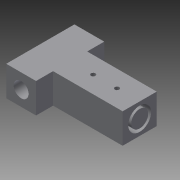
# Autodesk Inventor part: WagonHandleV01
Saved by Autodesk Inventor 2014 (Build 180170000, 170)
## iProperties
Created: 2013-11-15
Part Number: WagonHandleV01
Material: Generic
Document SubType Name: Modeling
Designer: steele
Density: 1 g/cm^3
Appearance: Default
Author: steele
Autodesk Inventor part; units mm, degrees
ref_plane "YZ Plane" through (0, 0, 0) normal (1, 0, 0) x (0, 1, 0)
ref_plane "XZ Plane" through (0, 0, 0) normal (0, 1, 0) x (-1, 0, 0)
sketch "Base for Part" plane through (0, 0, 0) normal (0, 0, 1) x (1, 0, 0)
  line L0 (0, 0) -> (148, 0) construction
  line L1 (0, 0) -> (0, 50.8)
  line L2 (0, 50.8) -> (44.45, 50.8)
  line L3 (148, -29.2) -> (148, 0)
  line L4 (44.45, 50.8) -> (44.45, 25.4)
  line L5 (44.45, 25.4) -> (148, 25.4)
  line L6 (148, 25.4) -> (148, 0)
  line L7 (0, 0) -> (0, -50.8)
  line L8 (0, -50.8) -> (44.45, -50.8)
  line L9 (44.45, -50.8) -> (44.45, -25.4)
  line L10 (44.45, -25.4) -> (148, -25.4)
  line L11 (148, -25.4) -> (148, 0)
  dimension "d0" = 148
  dimension "d1" = 50.8
  dimension "d2" = 44.45
  dimension "d3" = 25.4
  constraints: 24 end point, 4 perpendicular, 4 symmetric about line, 2 parallel
  measures "d0" distance of L0.start L0.end
  measures "d1" distance of L0.start L1.end
  measures "d2" distance of L1.end L2.end
  measures "d3" distance of L2.end L4.end
extrude "Extrusion of Base" add sketch "Base for Part" along normal blind 44.45
sketch "Sketch for 1 inch PVC" plane through (148, -25.4, 0) normal (1, 0, 0) x (0, 0, -1)
  line L0 (0, 50.8) -> (-44.45, 50.8) projected
  line L1 (-44.45, 0) -> (-44.45, 50.8) projected
  line L2 (0, 0) -> (-44.45, 0) projected
  line L3 (-44.45, 25.4) -> (0, 25.4) construction
  line L4 (-22.225, 50.8) -> (-22.225, 0) construction
  circle A0 centre (-22.225, 25.4) radius 12.6619
  circle A1 centre (-22.225, 25.4) radius 17.0434
  dimension "d6" = 34.0868
  dimension "d7" = 25.3238
  constraints: 4 end point, 4 midpoint, 2 centre point, 1 coincident, 1 parallel
  measures "d6" diameter of A1
  measures "d7" diameter of A0
extrude "Extrusion for 1 inch PVC" cut sketch "Sketch for 1 inch PVC" against normal blind 114.55
sketch "Sketch of Base Hole" plane through (0, -50.8, 0) normal (0, -1, 0) x (1, 0, 0)
  line L0 (44.45, 0) -> (0, 0) projected
  line L1 (44.45, 0) -> (44.45, 44.45) projected
  line L2 (0, 44.45) -> (44.45, 44.45) projected
  line L3 (0, 0) -> (0, 44.45) projected
  line L4 (0, 22.225) -> (44.45, 22.225) construction
  line L5 (22.225, 44.45) -> (22.225, 0) construction
  circle A0 centre (22.225, 22.225) radius 11.1506
  dimension "d10" = 22.3012
  constraints: 5 midpoint, 4 end point, 1 centre point
  measures "d10" diameter of A0
extrude "Extrusion3" cut sketch "Sketch of Base Hole" against normal through all contours A0
ref_plane "Work Plane1" through (0, 0, 44.45) normal (0, 0, 1) x (1, 0, 0)
sketch "Sketch9" plane through (0, 0, 44.45) normal (0, 0, 1) x (1, 0, 0)
  circle A0 centre (78.74, 0) radius 3.302
  circle A1 centre (114.3, 0) radius 3.302
  line L0 (149.86, 19.05) -> (149.86, -19.05) projected
  point P0 (0, 0)
  dimension "d39" = 6.604
  dimension "d42" = 35.56
  dimension "d43" = 71.12
  constraints: 2 centre point, 1 equal radius
  measures "d39" diameter of A0
  measures "d42" distance from line of A1.centre L0
  measures "d43" distance from line of L0 A0.centre
extrude "Extrusion6" cut sketch "Sketch9" against normal through all
body "Solid1"
